Autodesk Fusion 360 part; units mm, degrees
(part 2 of 2)
  spline S340 degree 2 poles (33.0314, 19.2318) (33.0668, 19.3037) (33.1231, 19.3533) knots 0 0 0 1 1 1
  spline S341 degree 2 poles (33.1231, 19.3533) (33.1795, 19.4029) (33.2488, 19.4303) knots 0 0 0 1 1 1
  spline S342 degree 2 poles (33.2488, 19.4303) (33.3182, 19.4576) (33.3835, 19.4575) knots 0 0 0 1 1 1
  spline S343 degree 2 poles (33.3835, 19.4575) (33.4829, 19.4574) (33.5627, 19.4206) knots 0 0 0 1 1 1
  spline S344 degree 2 poles (33.5627, 19.4206) (33.6424, 19.3839) (33.6998, 19.321) knots 0 0 0 1 1 1
  spline S345 degree 2 poles (33.6998, 19.321) (33.7573, 19.2582) (33.7872, 19.1757) knots 0 0 0 1 1 1
  spline S346 degree 2 poles (33.7872, 19.1757) (33.8172, 19.0933) (33.817, 19.0018) knots 0 0 0 1 1 1
  spline S347 degree 2 poles (33.817, 19.0018) (33.8168, 18.8762) (33.767, 18.7795) knots 0 0 0 1 1 1
  spline S348 degree 2 poles (33.767, 18.7795) (33.7172, 18.6828) (33.6321, 18.6176) knots 0 0 0 1 1 1
  spline S349 degree 2 poles (33.6321, 18.6176) (33.547, 18.5523) (33.4344, 18.5198) knots 0 0 0 1 1 1
  spline S350 degree 2 poles (33.4344, 18.5198) (33.3219, 18.4872) (33.1964, 18.4874) knots 0 0 0 1 1 1
  spline S351 degree 2 poles (33.1964, 18.4874) (33.0944, 18.4876) (32.961, 18.527) knots 0 0 0 1 1 1
  spline S352 degree 2 poles (32.961, 18.527) (32.8277, 18.5665) (32.6905, 18.6608) knots 0 0 0 1 1 1
  spline S353 degree 2 poles (32.6905, 18.6608) (32.5534, 18.7552) (32.4228, 18.9097) knots 0 0 0 1 1 1
  spline S354 degree 2 poles (32.4228, 18.9097) (32.2923, 19.0642) (32.1959, 19.2919) knots 0 0 0 1 1 1
  line L137 (32.1959, 19.2919) -> (32.1933, 17.6206)
  line L138 (32.1933, 17.6206) -> (33.8803, 17.6181)
  line L139 (33.8803, 17.6181) -> (34.0239, 17.4217)
  line L140 (34.0239, 17.4217) -> (31.5915, 17.4253)
  line L141 (31.5915, 17.4253) -> (31.4479, 17.6217)
  line L142 (30.488, 17.6232) -> (31.0242, 17.6224)
  line L143 (31.0242, 17.6224) -> (31.0283, 20.366)
  line L144 (31.0283, 20.366) -> (31.2373, 20.1774)
  line L145 (31.2373, 20.1774) -> (31.2341, 18.0667)
  spline S355 degree 2 poles (31.2341, 18.0667) (31.2341, 18.0327) (31.2679, 17.962) knots 0 0 0 1 1 1
  spline S356 degree 2 poles (31.2679, 17.962) (31.3018, 17.8913) (31.3501, 17.818) knots 0 0 0 1 1 1
  spline S357 degree 2 poles (31.3501, 17.818) (31.3984, 17.7447) (31.4545, 17.6871) knots 0 0 0 1 1 1
  spline S358 degree 2 poles (31.4545, 17.6871) (31.5107, 17.6295) (31.5551, 17.6216) knots 0 0 0 1 1 1
  line L146 (31.5551, 17.6216) -> (31.631, 17.6214)
  line L147 (31.631, 17.6214) -> (31.7745, 17.4251)
  line L148 (31.7745, 17.4251) -> (31.5862, 17.4253)
  spline S359 degree 2 poles (31.5862, 17.4253) (31.5209, 17.4411) (31.4738, 17.4687) knots 0 0 0 1 1 1
  spline S360 degree 2 poles (31.4738, 17.4687) (31.4268, 17.4962) (31.3876, 17.5381) knots 0 0 0 1 1 1
  spline S361 degree 2 poles (31.3876, 17.5381) (31.3485, 17.58) (31.3132, 17.6389) knots 0 0 0 1 1 1
  spline S362 degree 2 poles (31.3132, 17.6389) (31.278, 17.6978) (31.2337, 17.7764) knots 0 0 0 1 1 1
  line L149 (31.2337, 17.7764) -> (31.2324, 16.9159)
  spline S363 degree 2 poles (31.2324, 16.9159) (31.1827, 16.9395) (31.1501, 17.0049) knots 0 0 0 1 1 1
  spline S364 degree 2 poles (31.1501, 17.0049) (31.1175, 17.0703) (31.0954, 17.1488) knots 0 0 0 1 1 1
  spline S365 degree 2 poles (31.0954, 17.1488) (31.0733, 17.2273) (31.0577, 17.3032) knots 0 0 0 1 1 1
  spline S366 degree 2 poles (31.0577, 17.3032) (31.0421, 17.3791) (31.0265, 17.4262) knots 0 0 0 1 1 1
  line L150 (31.0265, 17.4262) -> (30.6316, 17.4268)
  line L151 (30.6316, 17.4268) -> (30.488, 17.6232)
  spline S367 degree 2 poles (50.2029, 44.0682) (49.9437, 44.0701) (49.6977, 44.2049) knots 0 0 0 1 1 1
  spline S368 degree 2 poles (49.6977, 44.2049) (49.4518, 44.3398) (49.3158, 44.5884) knots 0 0 0 1 1 1
  spline S369 degree 2 poles (49.3158, 44.5884) (49.1798, 44.837) (49.1818, 45.1057) knots 0 0 0 1 1 1
  spline S370 degree 2 poles (49.1818, 45.1057) (49.1838, 45.3718) (49.3213, 45.6163) knots 0 0 0 1 1 1
  spline S371 degree 2 poles (49.3213, 45.6163) (49.4589, 45.8609) (49.7047, 45.9948) knots 0 0 0 1 1 1
  spline S372 degree 2 poles (49.7047, 45.9948) (49.9506, 46.1288) (50.218, 46.1268) knots 0 0 0 1 1 1
  spline S373 degree 2 poles (50.218, 46.1268) (50.4854, 46.1248) (50.7293, 45.9873) knots 0 0 0 1 1 1
  spline S374 degree 2 poles (50.7293, 45.9873) (50.9731, 45.8498) (51.1078, 45.6032) knots 0 0 0 1 1 1
  spline S375 degree 2 poles (51.1078, 45.6032) (51.2424, 45.3566) (51.2404, 45.0906) knots 0 0 0 1 1 1
  spline S376 degree 2 poles (51.2404, 45.0906) (51.2384, 44.8219) (51.0982, 44.5753) knots 0 0 0 1 1 1
  spline S377 degree 2 poles (51.0982, 44.5753) (50.9579, 44.3287) (50.71, 44.1975) knots 0 0 0 1 1 1
  spline S378 degree 2 poles (50.71, 44.1975) (50.4621, 44.0663) (50.2029, 44.0682) knots 0 0 0 1 1 1
  spline S379 degree 2 poles (50.2041, 44.2387) (50.421, 44.2371) (50.6272, 44.3468) knots 0 0 0 1 1 1
  spline S380 degree 2 poles (50.6272, 44.3468) (50.8333, 44.4565) (50.9508, 44.6623) knots 0 0 0 1 1 1
  spline S381 degree 2 poles (50.9508, 44.6623) (51.0682, 44.8681) (51.0699, 45.0919) knots 0 0 0 1 1 1
  spline S382 degree 2 poles (51.0699, 45.0919) (51.0715, 45.3142) (50.9591, 45.519) knots 0 0 0 1 1 1
  spline S383 degree 2 poles (50.9591, 45.519) (50.8467, 45.7238) (50.6429, 45.8392) knots 0 0 0 1 1 1
  spline S384 degree 2 poles (50.6429, 45.8392) (50.4391, 45.9546) (50.2167, 45.9563) knots 0 0 0 1 1 1
  spline S385 degree 2 poles (50.2167, 45.9563) (49.9944, 45.9579) (49.7889, 45.8455) knots 0 0 0 1 1 1
  spline S386 degree 2 poles (49.7889, 45.8455) (49.5834, 45.7331) (49.4687, 45.53) knots 0 0 0 1 1 1
  spline S387 degree 2 poles (49.4687, 45.53) (49.354, 45.3269) (49.3523, 45.1045) knots 0 0 0 1 1 1
  spline S388 degree 2 poles (49.3523, 45.1045) (49.3507, 44.8808) (49.4645, 44.6732) knots 0 0 0 1 1 1
  spline S389 degree 2 poles (49.4645, 44.6732) (49.5782, 44.4657) (49.7834, 44.353) knots 0 0 0 1 1 1
  spline S390 degree 2 poles (49.7834, 44.353) (49.9886, 44.2403) (50.2041, 44.2387) knots 0 0 0 1 1 1
  line L152 (49.8815, 45.267) -> (49.7141, 45.3174)
  spline S391 degree 2 poles (49.7141, 45.3174) (49.7563, 45.4876) (49.89, 45.5883) knots 0 0 0 1 1 1
  spline S392 degree 2 poles (49.89, 45.5883) (50.0238, 45.6889) (50.2134, 45.6875) knots 0 0 0 1 1 1
  spline S393 degree 2 poles (50.2134, 45.6875) (50.4535, 45.6858) (50.6024, 45.5291) knots 0 0 0 1 1 1
  spline S394 degree 2 poles (50.6024, 45.5291) (50.7513, 45.3725) (50.7493, 45.097) knots 0 0 0 1 1 1
  spline S395 degree 2 poles (50.7493, 45.097) (50.748, 44.9169) (50.6788, 44.7844) knots 0 0 0 1 1 1
  spline S396 degree 2 poles (50.6788, 44.7844) (50.6096, 44.6519) (50.4829, 44.5853) knots 0 0 0 1 1 1
  spline S397 degree 2 poles (50.4829, 44.5853) (50.3562, 44.5187) (50.1939, 44.5198) knots 0 0 0 1 1 1
  spline S398 degree 2 poles (50.1939, 44.5198) (50.0125, 44.5212) (49.893, 44.6087) knots 0 0 0 1 1 1
  spline S399 degree 2 poles (49.893, 44.6087) (49.7736, 44.6962) (49.7311, 44.8452) knots 0 0 0 1 1 1
  line L153 (49.7311, 44.8452) -> (49.8937, 44.8836)
  spline S400 degree 2 poles (49.8937, 44.8836) (49.9339, 44.7823) (50.0133, 44.7279) knots 0 0 0 1 1 1
  spline S401 degree 2 poles (50.0133, 44.7279) (50.0927, 44.6734) (50.2005, 44.6726) knots 0 0 0 1 1 1
  spline S402 degree 2 poles (50.2005, 44.6726) (50.3574, 44.6714) (50.4598, 44.7826) knots 0 0 0 1 1 1
  spline S403 degree 2 poles (50.4598, 44.7826) (50.5623, 44.8937) (50.5638, 45.1024) knots 0 0 0 1 1 1
  spline S404 degree 2 poles (50.5638, 45.1024) (50.5654, 45.3111) (50.47, 45.4189) knots 0 0 0 1 1 1
  spline S405 degree 2 poles (50.47, 45.4189) (50.3746, 45.5267) (50.2218, 45.5279) knots 0 0 0 1 1 1
  spline S406 degree 2 poles (50.2218, 45.5279) (50.099, 45.5288) (50.0057, 45.4585) knots 0 0 0 1 1 1
  spline S407 degree 2 poles (50.0057, 45.4585) (49.9124, 45.3882) (49.8815, 45.267) knots 0 0 0 1 1 1
  line L154 (49.1971, 46.1098) -> (48.4144, 44.1155)
  line L155 (48.4144, 44.1155) -> (48.1293, 44.1175)
  line L156 (48.1293, 44.1175) -> (47.3254, 46.1235)
  line L157 (47.3254, 46.1235) -> (47.6269, 46.1213)
  line L158 (47.6269, 46.1213) -> (47.8557, 45.5139)
  line L159 (47.8557, 45.5139) -> (48.692, 45.5077)
  line L160 (48.692, 45.5077) -> (48.9161, 46.1118)
  line L161 (48.9161, 46.1118) -> (49.1971, 46.1098)
  line L162 (48.614, 45.2927) -> (47.936, 45.2977)
  line L163 (47.936, 45.2977) -> (48.1407, 44.7423)
  spline S408 degree 2 poles (48.1407, 44.7423) (48.2343, 44.4892) (48.2795, 44.3265) knots 0 0 0 1 1 1
  spline S409 degree 2 poles (48.2795, 44.3265) (48.3191, 44.5186) (48.3901, 44.7077) knots 0 0 0 1 1 1
  line L164 (48.3901, 44.7077) -> (48.614, 45.2927)
  spline S410 degree 2 poles (47.2312, 45.3998) (47.2282, 44.9973) (47.0031, 44.8052) knots 0 0 0 1 1 1
  spline S411 degree 2 poles (47.0031, 44.8052) (46.815, 44.6456) (46.5462, 44.6476) knots 0 0 0 1 1 1
  spline S412 degree 2 poles (46.5462, 44.6476) (46.2475, 44.6498) (46.0593, 44.847) knots 0 0 0 1 1 1
  spline S413 degree 2 poles (46.0593, 44.847) (45.8711, 45.0441) (45.8736, 45.3893) knots 0 0 0 1 1 1
  spline S414 degree 2 poles (45.8736, 45.3893) (45.8757, 45.6689) (45.9608, 45.8286) knots 0 0 0 1 1 1
  spline S415 degree 2 poles (45.9608, 45.8286) (46.0458, 45.9883) (46.2068, 46.0758) knots 0 0 0 1 1 1
  spline S416 degree 2 poles (46.2068, 46.0758) (46.3677, 46.1633) (46.5574, 46.1619) knots 0 0 0 1 1 1
  spline S417 degree 2 poles (46.5574, 46.1619) (46.8616, 46.1597) (47.0477, 45.9632) knots 0 0 0 1 1 1
  spline S418 degree 2 poles (47.0477, 45.9632) (47.2339, 45.7667) (47.2312, 45.3998) knots 0 0 0 1 1 1
  spline S419 degree 2 poles (46.9788, 45.4016) (46.9808, 45.6799) (46.8604, 45.8193) knots 0 0 0 1 1 1
  spline S420 degree 2 poles (46.8604, 45.8193) (46.74, 45.9586) (46.5559, 45.96) knots 0 0 0 1 1 1
  spline S421 degree 2 poles (46.5559, 45.96) (46.3731, 45.9613) (46.2506, 45.8231) knots 0 0 0 1 1 1
  spline S422 degree 2 poles (46.2506, 45.8231) (46.1282, 45.6848) (46.1261, 45.3997) knots 0 0 0 1 1 1
  spline S423 degree 2 poles (46.1261, 45.3997) (46.1241, 45.1309) (46.2452, 44.9916) knots 0 0 0 1 1 1
  spline S424 degree 2 poles (46.2452, 44.9916) (46.3663, 44.8522) (46.5477, 44.8509) knots 0 0 0 1 1 1
  spline S425 degree 2 poles (46.5477, 44.8509) (46.7319, 44.8495) (46.8543, 44.9864) knots 0 0 0 1 1 1
  spline S426 degree 2 poles (46.8543, 44.9864) (46.9767, 45.1233) (46.9788, 45.4016) knots 0 0 0 1 1 1
  line L165 (45.577, 44.4187) -> (45.5749, 44.1363)
  line L166 (45.5749, 44.1363) -> (45.3294, 44.1381)
  line L167 (45.3294, 44.1381) -> (45.3315, 44.4205)
  line L168 (45.3315, 44.4205) -> (45.577, 44.4187)
  line L169 (45.5896, 46.1363) -> (45.579, 44.6875)
  line L170 (45.579, 44.6875) -> (45.3334, 44.6893)
  line L171 (45.3334, 44.6893) -> (45.3441, 46.1381)
  line L172 (45.3441, 46.1381) -> (45.5896, 46.1363)
  line L173 (45.0651, 45.7076) -> (44.822, 45.6712)
  spline S427 degree 2 poles (44.822, 45.6712) (44.8026, 45.8173) (44.7097, 45.8958) knots 0 0 0 1 1 1
  spline S428 degree 2 poles (44.7097, 45.8958) (44.6168, 45.9742) (44.449, 45.9755) knots 0 0 0 1 1 1
  spline S429 degree 2 poles (44.449, 45.9755) (44.2799, 45.9767) (44.1975, 45.9084) knots 0 0 0 1 1 1
  spline S430 degree 2 poles (44.1975, 45.9084) (44.1151, 45.8401) (44.1145, 45.7474) knots 0 0 0 1 1 1
  spline S431 degree 2 poles (44.1145, 45.7474) (44.1139, 45.6642) (44.1858, 45.6159) knots 0 0 0 1 1 1
  spline S432 degree 2 poles (44.1858, 45.6159) (44.236, 45.5828) (44.4362, 45.5308) knots 0 0 0 1 1 1
  spline S433 degree 2 poles (44.4362, 45.5308) (44.7058, 45.4606) (44.8098, 45.4101) knots 0 0 0 1 1 1
  spline S434 degree 2 poles (44.8098, 45.4101) (44.9138, 45.3595) (44.9671, 45.2711) knots 0 0 0 1 1 1
  spline S435 degree 2 poles (44.9671, 45.2711) (45.0203, 45.1827) (45.0195, 45.0763) knots 0 0 0 1 1 1
  spline S436 degree 2 poles (45.0195, 45.0763) (45.0188, 44.9794) (44.9739, 44.8972) knots 0 0 0 1 1 1
  spline S437 degree 2 poles (44.9739, 44.8972) (44.9289, 44.815) (44.8521, 44.761) knots 0 0 0 1 1 1
  spline S438 degree 2 poles (44.8521, 44.761) (44.7945, 44.7192) (44.6954, 44.6905) knots 0 0 0 1 1 1
  spline S439 degree 2 poles (44.6954, 44.6905) (44.5963, 44.6619) (44.483, 44.6628) knots 0 0 0 1 1 1
  spline S440 degree 2 poles (44.483, 44.6628) (44.3125, 44.664) (44.184, 44.7141) knots 0 0 0 1 1 1
  spline S441 degree 2 poles (44.184, 44.7141) (44.0554, 44.7641) (43.9946, 44.8485) knots 0 0 0 1 1 1
  spline S442 degree 2 poles (43.9946, 44.8485) (43.9338, 44.9328) (43.9117, 45.0735) knots 0 0 0 1 1 1
  line L174 (43.9117, 45.0735) -> (44.152, 45.1045)
  spline S443 degree 2 poles (44.152, 45.1045) (44.1676, 44.9925) (44.2456, 44.9292) knots 0 0 0 1 1 1
  spline S444 degree 2 poles (44.2456, 44.9292) (44.3235, 44.8659) (44.4668, 44.8648) knots 0 0 0 1 1 1
  spline S445 degree 2 poles (44.4668, 44.8648) (44.6359, 44.8636) (44.7087, 44.919) knots 0 0 0 1 1 1
  spline S446 degree 2 poles (44.7087, 44.919) (44.7814, 44.9744) (44.7819, 45.0494) knots 0 0 0 1 1 1
  spline S447 degree 2 poles (44.7819, 45.0494) (44.7823, 45.0971) (44.7525, 45.1356) knots 0 0 0 1 1 1
  spline S448 degree 2 poles (44.7525, 45.1356) (44.7228, 45.1754) (44.6589, 45.2017) knots 0 0 0 1 1 1
  spline S449 degree 2 poles (44.6589, 45.2017) (44.6222, 45.2157) (44.4424, 45.2661) knots 0 0 0 1 1 1
  spline S450 degree 2 poles (44.4424, 45.2661) (44.1824, 45.3376) (44.0797, 45.3827) knots 0 0 0 1 1 1
  spline S451 degree 2 poles (44.0797, 45.3827) (43.977, 45.4278) (43.919, 45.5128) knots 0 0 0 1 1 1
  spline S452 degree 2 poles (43.919, 45.5128) (43.861, 45.5978) (43.8619, 45.7233) knots 0 0 0 1 1 1
  spline S453 degree 2 poles (43.8619, 45.7233) (43.8628, 45.8461) (43.9352, 45.954) knots 0 0 0 1 1 1
  spline S454 degree 2 poles (43.9352, 45.954) (44.0076, 46.0619) (44.1431, 46.1203) knots 0 0 0 1 1 1
  spline S455 degree 2 poles (44.1431, 46.1203) (44.2786, 46.1786) (44.4491, 46.1774) knots 0 0 0 1 1 1
  spline S456 degree 2 poles (44.4491, 46.1774) (44.7315, 46.1753) (44.8787, 46.0569) knots 0 0 0 1 1 1
  spline S457 degree 2 poles (44.8787, 46.0569) (45.0259, 45.9385) (45.0651, 45.7076) knots 0 0 0 1 1 1
  line L175 (43.5728, 46.1511) -> (43.5581, 44.1511)
  line L176 (43.5581, 44.1511) -> (43.3126, 44.1529)
  line L177 (43.3126, 44.1529) -> (43.3178, 44.8705)
  spline S458 degree 2 poles (43.3178, 44.8705) (43.1445, 44.6726) (42.8826, 44.6745) knots 0 0 0 1 1 1
  spline S459 degree 2 poles (42.8826, 44.6745) (42.7216, 44.6757) (42.6034, 44.74) knots 0 0 0 1 1 1
  spline S460 degree 2 poles (42.6034, 44.74) (42.4851, 44.8043) (42.4348, 44.9166) knots 0 0 0 1 1 1
  spline S461 degree 2 poles (42.4348, 44.9166) (42.3845, 45.0288) (42.386, 45.2416) knots 0 0 0 1 1 1
  line L178 (42.386, 45.2416) -> (42.3928, 46.1598)
  line L179 (42.3928, 46.1598) -> (42.6383, 46.158)
  line L180 (42.6383, 46.158) -> (42.6316, 45.2398)
  spline S462 degree 2 poles (42.6316, 45.2398) (42.6302, 45.0557) (42.7094, 44.9712) knots 0 0 0 1 1 1
  spline S463 degree 2 poles (42.7094, 44.9712) (42.7886, 44.8867) (42.9346, 44.8856) knots 0 0 0 1 1 1
  spline S464 degree 2 poles (42.9346, 44.8856) (43.0437, 44.8848) (43.1403, 44.9407) knots 0 0 0 1 1 1
  spline S465 degree 2 poles (43.1403, 44.9407) (43.2369, 44.9966) (43.2786, 45.0932) knots 0 0 0 1 1 1
  spline S466 degree 2 poles (43.2786, 45.0932) (43.3202, 45.1898) (43.3214, 45.3603) knots 0 0 0 1 1 1
  line L181 (43.3214, 45.3603) -> (43.3273, 46.1529)
  line L182 (43.3273, 46.1529) -> (43.5728, 46.1511)
  line L183 (42.0048, 44.445) -> (42.0027, 44.1626)
  line L184 (42.0027, 44.1626) -> (41.7571, 44.1644)
  line L185 (41.7571, 44.1644) -> (41.7592, 44.4468)
  line L186 (41.7592, 44.4468) -> (42.0048, 44.445)
  line L187 (42.0174, 46.1625) -> (42.0067, 44.7137)
  line L188 (42.0067, 44.7137) -> (41.7612, 44.7155)
  line L189 (41.7612, 44.7155) -> (41.7718, 46.1643)
  line L190 (41.7718, 46.1643) -> (42.0174, 46.1625)
  line L191 (41.3964, 46.1671) -> (41.3817, 44.1671)
  line L192 (41.3817, 44.1671) -> (41.1361, 44.1689)
  line L193 (41.1361, 44.1689) -> (41.1445, 45.3094)
  line L194 (41.1445, 45.3094) -> (40.559, 44.7244)
  line L195 (40.559, 44.7244) -> (40.2412, 44.7267)
  line L196 (40.2412, 44.7267) -> (40.799, 45.2601)
  line L197 (40.799, 45.2601) -> (40.1959, 46.1759)
  line L198 (40.1959, 46.1759) -> (40.4988, 46.1737)
  line L199 (40.4988, 46.1737) -> (40.9721, 45.4294)
  line L200 (40.9721, 45.4294) -> (41.1466, 45.5946)
  line L201 (41.1466, 45.5946) -> (41.1508, 46.1689)
  line L202 (41.1508, 46.1689) -> (41.3964, 46.1671)
  line L203 (39.2036, 46.1832) -> (39.1889, 44.1833)
  line L204 (39.1889, 44.1833) -> (38.9243, 44.1852)
  line L205 (38.9243, 44.1852) -> (38.9315, 45.177)
  line L206 (38.9315, 45.177) -> (37.9311, 44.1925)
  line L207 (37.9311, 44.1925) -> (37.5723, 44.1951)
  line L208 (37.5723, 44.1951) -> (38.4173, 44.9993)
  line L209 (38.4173, 44.9993) -> (37.5502, 46.1954)
  line L210 (37.5502, 46.1954) -> (37.8994, 46.1928)
  line L211 (37.8994, 46.1928) -> (38.6041, 45.1753)
  line L212 (38.6041, 45.1753) -> (38.9339, 45.4921)
  line L213 (38.9339, 45.4921) -> (38.939, 46.1851)
  line L214 (38.939, 46.1851) -> (39.2036, 46.1832)
  line L215 (37.3603, 46.1967) -> (37.3456, 44.1968)
  line L216 (37.3456, 44.1968) -> (37.1, 44.1986)
  line L217 (37.1, 44.1986) -> (37.1053, 44.9162)
  spline S467 degree 2 poles (37.1053, 44.9162) (36.932, 44.7183) (36.67, 44.7202) knots 0 0 0 1 1 1
  spline S468 degree 2 poles (36.67, 44.7202) (36.5091, 44.7214) (36.3908, 44.7857) knots 0 0 0 1 1 1
  spline S469 degree 2 poles (36.3908, 44.7857) (36.2726, 44.85) (36.2223, 44.9622) knots 0 0 0 1 1 1
  spline S470 degree 2 poles (36.2223, 44.9622) (36.1719, 45.0745) (36.1735, 45.2873) knots 0 0 0 1 1 1
  line L218 (36.1735, 45.2873) -> (36.1803, 46.2054)
  line L219 (36.1803, 46.2054) -> (36.4258, 46.2036)
  line L220 (36.4258, 46.2036) -> (36.4191, 45.2855)
  spline S471 degree 2 poles (36.4191, 45.2855) (36.4177, 45.1013) (36.4969, 45.0168) knots 0 0 0 1 1 1
  spline S472 degree 2 poles (36.4969, 45.0168) (36.5761, 44.9324) (36.7221, 44.9313) knots 0 0 0 1 1 1
  spline S473 degree 2 poles (36.7221, 44.9313) (36.8312, 44.9305) (36.9278, 44.9864) knots 0 0 0 1 1 1
  spline S474 degree 2 poles (36.9278, 44.9864) (37.0244, 45.0423) (37.066, 45.1389) knots 0 0 0 1 1 1
  spline S475 degree 2 poles (37.066, 45.1389) (37.1077, 45.2354) (37.1089, 45.4059) knots 0 0 0 1 1 1
  line L221 (37.1089, 45.4059) -> (37.1147, 46.1986)
  line L222 (37.1147, 46.1986) -> (37.3603, 46.1967)
  spline S476 degree 2 poles (34.8595, 46.0364) (34.9968, 46.1514) (35.1233, 46.1982) knots 0 0 0 1 1 1
  spline S477 degree 2 poles (35.1233, 46.1982) (35.2499, 46.245) (35.3945, 46.2439) knots 0 0 0 1 1 1
  spline S478 degree 2 poles (35.3945, 46.2439) (35.6332, 46.2422) (35.7606, 46.1246) knots 0 0 0 1 1 1
  spline S479 degree 2 poles (35.7606, 46.1246) (35.888, 46.007) (35.8866, 45.8256) knots 0 0 0 1 1 1
  spline S480 degree 2 poles (35.8866, 45.8256) (35.8858, 45.7192) (35.8368, 45.6315) knots 0 0 0 1 1 1
  spline S481 degree 2 poles (35.8368, 45.6315) (35.7877, 45.5439) (35.7089, 45.4913) knots 0 0 0 1 1 1
  spline S482 degree 2 poles (35.7089, 45.4913) (35.63, 45.4386) (35.5316, 45.4121) knots 0 0 0 1 1 1
  spline S483 degree 2 poles (35.5316, 45.4121) (35.4592, 45.3935) (35.3131, 45.3768) knots 0 0 0 1 1 1
  spline S484 degree 2 poles (35.3131, 45.3768) (35.0154, 45.3436) (34.8745, 45.2955) knots 0 0 0 1 1 1
  spline S485 degree 2 poles (34.8745, 45.2955) (34.8728, 45.245) (34.8727, 45.2314) knots 0 0 0 1 1 1
  spline S486 degree 2 poles (34.8727, 45.2314) (34.8716, 45.0813) (34.9407, 45.0194) knots 0 0 0 1 1 1
  spline S487 degree 2 poles (34.9407, 45.0194) (35.0342, 44.9355) (35.2198, 44.9341) knots 0 0 0 1 1 1
  spline S488 degree 2 poles (35.2198, 44.9341) (35.393, 44.9329) (35.476, 44.993) knots 0 0 0 1 1 1
  spline S489 degree 2 poles (35.476, 44.993) (35.559, 45.0531) (35.5997, 45.2069) knots 0 0 0 1 1 1
  line L223 (35.5997, 45.2069) -> (35.8395, 45.1724)
  spline S490 degree 2 poles (35.8395, 45.1724) (35.8057, 45.0185) (35.7299, 44.9242) knots 0 0 0 1 1 1
  spline S491 degree 2 poles (35.7299, 44.9242) (35.6542, 44.83) (35.5119, 44.7799) knots 0 0 0 1 1 1
  spline S492 degree 2 poles (35.5119, 44.7799) (35.3697, 44.7298) (35.1828, 44.7311) knots 0 0 0 1 1 1
  spline S493 degree 2 poles (35.1828, 44.7311) (34.9973, 44.7325) (34.8816, 44.777) knots 0 0 0 1 1 1
  spline S494 degree 2 poles (34.8816, 44.777) (34.766, 44.8215) (34.7119, 44.8881) knots 0 0 0 1 1 1
  spline S495 degree 2 poles (34.7119, 44.8881) (34.6578, 44.9546) (34.6367, 45.0557) knots 0 0 0 1 1 1
  spline S496 degree 2 poles (34.6367, 45.0557) (34.6249, 45.1186) (34.6261, 45.2823) knots 0 0 0 1 1 1
  line L224 (34.6261, 45.2823) -> (34.6285, 45.6097)
  spline S497 degree 2 poles (34.6285, 45.6097) (34.631, 45.9521) (34.616, 46.043) knots 0 0 0 1 1 1
  spline S498 degree 2 poles (34.616, 46.043) (34.601, 46.1338) (34.5552, 46.2174) knots 0 0 0 1 1 1
  line L225 (34.5552, 46.2174) -> (34.8117, 46.2155)
  spline S499 degree 2 poles (34.8117, 46.2155) (34.8493, 46.1388) (34.8595, 46.0364) knots 0 0 0 1 1 1
  spline S500 degree 2 poles (34.8759, 45.4878) (35.01, 45.5414) (35.2777, 45.5777) knots 0 0 0 1 1 1
  spline S501 degree 2 poles (35.2777, 45.5777) (35.4293, 45.5984) (35.4922, 45.6252) knots 0 0 0 1 1 1
  spline S502 degree 2 poles (35.4922, 45.6252) (35.5552, 45.652) (35.5897, 45.7043) knots 0 0 0 1 1 1
  spline S503 degree 2 poles (35.5897, 45.7043) (35.6242, 45.7566) (35.6246, 45.8207) knots 0 0 0 1 1 1
  spline S504 degree 2 poles (35.6246, 45.8207) (35.6254, 45.9189) (35.5515, 45.9849) knots 0 0 0 1 1 1
  spline S505 degree 2 poles (35.5515, 45.9849) (35.4776, 46.051) (35.3344, 46.052) knots 0 0 0 1 1 1
  spline S506 degree 2 poles (35.3344, 46.052) (35.1925, 46.0531) (35.0815, 45.9918) knots 0 0 0 1 1 1
  spline S507 degree 2 poles (35.0815, 45.9918) (34.9706, 45.9305) (34.918, 45.8231) knots 0 0 0 1 1 1
  spline S508 degree 2 poles (34.918, 45.8231) (34.8778, 45.7402) (34.8766, 45.5779) knots 0 0 0 1 1 1
  line L226 (34.8766, 45.5779) -> (34.8759, 45.4878)
  line L227 (34.2521, 46.2196) -> (34.2415, 44.7708)
  line L228 (34.2415, 44.7708) -> (34.0205, 44.7724)
  line L229 (34.0205, 44.7724) -> (34.022, 44.9784)
  spline S509 degree 2 poles (34.022, 44.9784) (33.8606, 44.7408) (33.5591, 44.7431) knots 0 0 0 1 1 1
  spline S510 degree 2 poles (33.5591, 44.7431) (33.4282, 44.744) (33.3187, 44.7919) knots 0 0 0 1 1 1
  spline S511 degree 2 poles (33.3187, 44.7919) (33.2092, 44.8398) (33.1552, 44.9166) knots 0 0 0 1 1 1
  spline S512 degree 2 poles (33.1552, 44.9166) (33.1012, 44.9934) (33.0801, 45.0986) knots 0 0 0 1 1 1
  spline S513 degree 2 poles (33.0801, 45.0986) (33.067, 45.1669) (33.0683, 45.3374) knots 0 0 0 1 1 1
  line L230 (33.0683, 45.3374) -> (33.0748, 46.2282)
  line L231 (33.0748, 46.2282) -> (33.3204, 46.2264)
  line L232 (33.3204, 46.2264) -> (33.3139, 45.3452)
  spline S514 degree 2 poles (33.3139, 45.3452) (33.3128, 45.1951) (33.3409, 45.1205) knots 0 0 0 1 1 1
  spline S515 degree 2 poles (33.3409, 45.1205) (33.369, 45.046) (33.4416, 45.0011) knots 0 0 0 1 1 1
  spline S516 degree 2 poles (33.4416, 45.0011) (33.5143, 44.9562) (33.6125, 44.9555) knots 0 0 0 1 1 1
  spline S517 degree 2 poles (33.6125, 44.9555) (33.7694, 44.9543) (33.8841, 45.0531) knots 0 0 0 1 1 1
  spline S518 degree 2 poles (33.8841, 45.0531) (33.9987, 45.1518) (34.0007, 45.4301) knots 0 0 0 1 1 1
  line L233 (34.0007, 45.4301) -> (34.0066, 46.2214)
  line L234 (34.0066, 46.2214) -> (34.2521, 46.2196)
extrude "Extrude2" cut sketch "Sketch2" against normal blind 0.8 contours L0 L1 S0 S1 S2 S3 S4 S5 S6 S7 S8 L2 | S16 S17 S18 S19 S20 S21 S22 S23 S24 S25 S26 | L6 L7 L8 L9 L10 L11 L12 L13 L14 L15 | S36 S37 S38 S39 S40 S41 S42 S43 S44 S45 S46 | L16 L17 L18 L19 L20 L21 L22 L23 | L24 L25 L26 L27 L28 L29 L30 L31 | S56 S57 S58 S59 S60 S61 S62 S63 S64 S65 S66 | L32 L33 S76 S77 S78 S79 S80 S81 L34 L35 L36 S82 S83 S84 S85 S86 L37 | L38 S87 S88 S89 S90 S91 S92 S93 S94 S95 S96 L39 S97 S98 S99 S100 S101 S102 S103 S104 S105 S106 | L40 L41 L42 L43 L44 L45 L46 L47 L48 L49 L50 L51 | L66 L69 L70 L71 L72 S173 S174 S175 S176 S177 S178 S179 S180 S181 S182 S183 S184 S185 S186 S187 S188 S189 S190 S191 S192 S193 S194 S195 S196 S197 S198 S199 S200 S201 S202 S203 S204 L73 L75 S205 S206 S207 S208 S209 S210 S211 S212 S213 S214 L76 S217 S218 L77 L78 L80 | L52 L53 L54 L55 S107 S108 S109 S110 L56 L57 S111 S112 S113 S114 S115 S116 S117 S118 S119 S120 S121 S122 S123 S124 S125 S126 S127 S128 S129 S130 L58 S131 S132 S133 S134 S135 S136 S137 S138 L59 L60 L61 L62 L63 S139 S140 S141 S142 S143 S144 L64 S145 S146 S147 S148 L65 L74 | S215 S216 S217 L79 L80 L81 L82 | L94 L97 L98 L99 S249 S250 S251 S252 L100 L101 L102 L103 L105 L111 | L83 L84 S219 S220 S221 S222 S223 S224 S225 S226 S227 S228 S229 S230 S231 S232 S233 S234 S235 S236 S237 S238 S239 S240 L85 L86 L87 S241 S242 S243 S244 L88 L89 L90 L91 L92 L93 L104 | L106 L109 S265 S266 S267 S268 S269 S270 S271 S272 S273 S274 S275 S276 S277 S278 S279 S280 S281 S282 S283 S284 S285 S286 S287 S288 S289 S290 S291 S292 S293 S294 S295 S296 S297 S298 S299 S300 L110 L112 L121 | L113 L114 L115 L116 S301 S302 S303 S304 L117 L118 L119 L120 L122 L131 | L123 L126 L127 L128 S309 S310 S311 S312 S313 S314 S315 S316 S317 S318 S319 S320 S321 S322 S323 S324 S325 S326 S327 S328 S329 S330 S331 L129 L130 L132 L133 | S257 S258 S259 S260 S261 S262 S263 S264 | L134 L141 L142 L143 L144 L145 S355 S356 S357 S358 L148 S359 S360 S361 S362 L149 S363 S364 S365 S366 L150 L151 | L134 L135 L136 S332 S333 S334 S335 S336 S337 S338 S339 S340 S341 S342 S343 S344 S345 S346 S347 S348 S349 S350 S351 S352 S353 S354 L137 L138 L139 L140 L147 | S379 S380 S381 S382 S383 S384 S385 S386 S387 S388 S389 S390 | L154 L155 L156 L157 L158 L159 L160 L161 | S410 S411 S412 S413 S414 S415 S416 S417 S418 | L165 L166 L167 L168 | L169 L170 L171 L172 | L173 S427 S428 S429 S430 S431 S432 S433 S434 S435 S436 S437 S438 S439 S440 S441 S442 L174 S443 S444 S445 S446 S447 S448 S449 S450 S451 S452 S453 S454 S455 S456 S457 | L175 L176 L177 S458 S459 S460 S461 L178 L179 L180 S462 S463 S464 S465 S466 L181 L182 | L183 L184 L185 L186 | L187 L188 L189 L190 | L191 L192 L193 L194 L195 L196 L197 L198 L199 L200 L201 L202 | L203 L204 L205 L206 L207 L208 L209 L210 L211 L212 L213 L214 | L215 L216 L217 S467 S468 S469 S470 L218 L219 L220 S471 S472 S473 S474 S475 L221 L222 | S476 S477 S478 S479 S480 S481 S482 S483 S484 S485 S486 S487 S488 S489 L223 S490 S491 S492 S493 S494 S495 S496 L224 S497 S498 L225 S499 | L227 L228 L229 S509 S510 S511 S512 S513 L230 L231 L232 S514 S515 S516 S517 S518 L233 L234
fillet "Fillet1" radius 5 4 edges at (20.1962, 5, 0.875) (64.1962, 5, 0.875) (64.1962, 49, 0.875) (20.1962, 49, 0.875)
fillet "Fillet2" radius 2 8 edges at (62.7317, 6.4645, 1.75) (64.1962, 27, 1.75) (62.7317, 47.5355, 1.75) (42.1962, 49, 1.75) (21.6606, 47.5355, 1.75) (20.1962, 27, 1.75) (21.6606, 6.4645, 1.75) (42.1962, 5, 1.75)
